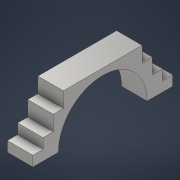
# Autodesk Inventor part: 110033226_ipt_03_小橋
Saved by Autodesk Inventor 2022 (Build 260153000, 153)
## iProperties
Created: 2022-06-22
Part Number: 110033226_ipt_03_小橋
Material: 一般
Document SubType Name: Modeling
Designer: User
Density: 1 g/cm^3
Appearance: 預設
Author: User
Autodesk Inventor part; units mm, degrees
ref_plane "XZ Plane" through (0, 0, 0) normal (0, 1, 0) x (-1, 0, 0)
ref_plane "XY Plane" through (0, 0, 0) normal (0, 0, 1) x (1, 0, 0)
sketch "草圖1" plane through (0, 0, 0) normal (0, 1, 0) x (-1, 0, 0)
  line L0 (5, 27.5) -> (-5, 27.5)
  line L1 (-5, 27.5) -> (-5, -27.5)
  line L2 (-5, -27.5) -> (5, -27.5)
  line L3 (5, -27.5) -> (5, 27.5)
  circle A0 centre (2.5, 25) radius 1.7
  circle A1 centre (2.5, 20) radius 1.7
  circle A2 centre (-2.5, 25) radius 1.7
  circle A3 centre (-2.5, 20) radius 1.7
  line L4 (5, 17.5) -> (-5, 17.5)
  line L5 (5, 0) -> (-5, 0) construction
  circle A4 centre (2.5, -25) radius 1.7
  circle A5 centre (2.5, -20) radius 1.7
  circle A6 centre (-2.5, -25) radius 1.7
  circle A7 centre (-2.5, -20) radius 1.7
  line L6 (5, -17.5) -> (-5, -17.5)
  point P0 (0, 0)
  point P1 (0, -27.5)
  dimension "d0" = 10
  dimension "d1" = 55
  dimension "d2" = 3.4
  dimension "d3" = 2.5
  dimension "d4" = 2.5
  dimension "d7" = 5
  dimension "d10" = 5
  dimension "d13" = 2.5
  constraints: 14 end point, 8 centre point, 6 symmetric about line, 3 midpoint, 2 horizontal, 2 parallel, 2 perpendicular, 2 point on line, 1 horizontal alignment, 1 vertical, 1 vertical alignment, 10 other
  measures "d0" distance of L2.end L1.end
  measures "d1" distance of L1.end L0.end
  measures "d2" diameter of A0
  measures "d3" distance from line of L3 A0.centre
  measures "d4" distance from line of L0 A0.centre
  measures "d7" distance of A0.centre A1.centre
  measures "d10" distance of A0.centre A2.centre
  measures "d13" distance from line of A1.centre L4
ref_plane "工作平面1" through (5, 0, 0) normal (1, 0, 0) x (0, 1, 0)
sketch "草圖2" plane through (5, 0, 0) normal (1, 0, 0) x (0, 1, 0)
  line L0 (0, 27.5) -> (0, -27.5) projected
  arc A0 (0, -17.5) -> (0, 17.5) centre (0, 0) ccw
  line L1 (0, 27.5) -> (4, 27.5)
  line L2 (4, 27.5) -> (4, 23.5)
  line L3 (4, 23.5) -> (8, 23.5)
  line L4 (8, 23.5) -> (8, 19.5)
  line L5 (8, 19.5) -> (14, 19.5)
  line L6 (14, 19.5) -> (14, 15.5)
  line L7 (14, 15.5) -> (20, 15.5)
  line L8 (20, 15.5) -> (20, 0)
  line L9 (17.5, 0) -> (0, 0) construction
  line L10 (0, -27.5) -> (4, -27.5)
  line L11 (4, -27.5) -> (4, -23.5)
  line L12 (4, -23.5) -> (8, -23.5)
  line L13 (8, -23.5) -> (8, -19.5)
  line L14 (8, -19.5) -> (14, -19.5)
  line L15 (14, -19.5) -> (14, -15.5)
  line L16 (14, -15.5) -> (20, -15.5)
  line L17 (20, -15.5) -> (20, 0)
  dimension "d14" = 4
  dimension "d15" = 4
  dimension "d16" = 4
  dimension "d17" = 4
  dimension "d18" = 6
  dimension "d19" = 4
  dimension "d21" = 6
  constraints: 34 end point, 7 symmetric about line, 6 perpendicular, 4 point on circle, 3 horizontal, 2 point on line, 1 centre point, 1 coincident
  measures "d14" distance of L0.start L1.end
  measures "d15" distance of L1.end L2.end
  measures "d16" distance of L2.end L3.end
  measures "d17" distance of L3.end L4.end
  measures "d18" distance of L4.end L5.end
  measures "d19" distance of L5.end L6.end
  measures "d21" distance of L6.end L7.end
extrude "擠出1" add sketch "草圖2" against normal blind 10 contours L1 L2 L3 L4 L5 L6 L7 L8 L17 L16 L15 L14 L13 L12 L11 L10 L0 A0
extrude "擠出2" cut sketch "草圖1" along normal blind 1.5 contours A0 | A1 | A2 | A3 | A4 | A5 | A6 | A7
